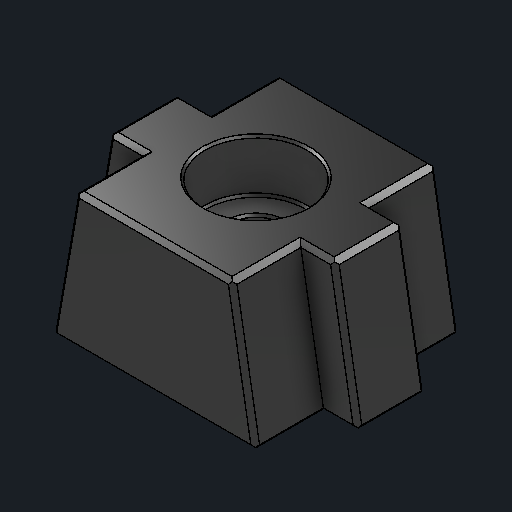
# Autodesk Inventor part: 4 Way Fixture Base
Saved by Autodesk Inventor 2026.2 (Build 302298000, 298)
## iProperties
Created: 2026-05-18
Part Number: 4 Way Fixture Base
Material: ABS Plastic
Document SubType Name: Modeling
Designer: JoshuaEah
Density: 1.06 g/cm^3
Appearance: Glossy - Black
Author: JoshuaEah
Autodesk Inventor part; units mm, degrees
ref_plane "YZ Plane" through (0, 0, 0) normal (1, 0, 0) x (0, 1, 0)
ref_plane "XZ Plane" through (0, 0, 0) normal (0, 1, 0) x (-1, 0, 0)
ref_plane "XY Plane" through (0, 0, 0) normal (0, 0, 1) x (1, 0, 0)
sketch "Sketch4" plane through (0, 0, 0) normal (0, 1, 0) x (-1, 0, 0)
  line L0 (0, 0) -> (-25.4, 0)
  line L1 (-25.4, 0) -> (-25.4, -19.05)
  line L2 (-25.4, -19.05) -> (0, -19.05)
  line L3 (0, -19.05) -> (0, 0)
  line L4 (0, -9.525) -> (-25.4, -9.525) construction
  circle A0 centre (-12.7, -9.525) radius 3.175
  line L5 (-3.175, -19.05) -> (-3.175, 0)
  line L6 (-12.7, -19.05) -> (-12.7, 0) construction
  line L7 (-22.225, -19.05) -> (-22.225, 0)
  line L8 (0, -12.7) -> (-3.175, -12.7)
  line L9 (0, -6.35) -> (-3.175, -6.35)
  line L10 (-25.4, -12.7) -> (-22.225, -12.7)
  line L11 (-25.4, -6.35) -> (-22.225, -6.35)
  point P0 (-25.4, -6.35)
  point P1 (-22.225, -6.35)
  point P2 (-22.225, 0)
  point P3 (-25.4, -12.7)
  point P4 (-22.225, -19.05)
  point P5 (-3.175, -6.35)
  point P6 (0, -6.35)
  dimension "d35" = 25.4
  dimension "d36" = 19.05
  dimension "d37" = 6.35
  dimension "d39" = 3.175
  dimension "d46" = 6.35
  constraints: 24 end point, 8 symmetric about line, 5 midpoint, 4 point on line, 2 horizontal, 2 parallel, 2 perpendicular, 1 centre point, 1 coincident, 1 vertical
  measures "d35" distance of L2.end L1.end
  measures "d36" distance of L1.end L0.end
  measures "d37" diameter of A0
  measures "d39" distance between parallel lines of L3 L5
  measures "d46" diameter of L8 L4
extrude "Extrusion5" add sketch "Sketch4" against normal blind 12.7 contours L3 L9 L5 L0 | L5 L2 L7 L0 | L3 L8 L5 L9 | L7 L11 L1 L0 | L3 L2 L5 L8 | L7 L10 L1 L11 | L7 L2 L1 L10 | A0
extrude "Extrusion6" cut sketch "Sketch4" against normal blind 12.7 contours L3 L9 L5 L0 | L7 L11 L1 L0 | L3 L2 L5 L8 | L7 L2 L1 L10
hole "Hole3" at (12.7, 0, -9.525) direction (0, -1, 0) diameter 5.1054 end through all counterbore diameter 9.525 counterbore depth 4.826 clearance for "Socket Head Cap Screw" size "#10" standard "Ansi Unified Screw Threads"
draft "FaceDraft2" angle 10 pull direction (0, 1, 0) faces at (25.4, -4.2333, -8.4667) (22.225, -4.2333, -16.9333) (22.225, -4.2333, -4.2333) (3.175, -4.2333, -2.1167) (0, -4.2333, -10.5833) (3.175, -4.2333, -14.8167) fixed edges at (25.4, -12.7, -9.525) (22.225, -12.7, -15.875) (22.225, -12.7, -3.175) (3.175, -12.7, -3.175) (3.175, -12.7, -15.875) (0, -12.7, -9.525)
chamfer "Chamfer1" distance 0.4 angle 45 32 edges at (12.7, 0, 0) (2.2394, 0, -9.525) (19.9856, 0, -3.175) (3.8269, 0, -6.35) (5.4144, 0, -3.175) (3.8269, 0, -12.7) (19.9856, 0, -15.875) (5.4144, 0, -15.875) (12.7, 0, -19.05) (21.5731, 0, -12.7) (23.1606, 0, -9.525) (21.5731, 0, -6.35) (3.175, -12.7, -3.175) (1.5875, -12.7, -6.35) (0, -12.7, -9.525) (1.5875, -12.7, -12.7) (3.175, -12.7, -15.875) (12.7, -12.7, -19.05) (22.225, -12.7, -15.875) (23.8125, -12.7, -12.7) (25.4, -12.7, -9.525) (23.8125, -12.7, -6.35) (22.225, -12.7, -3.175) (12.7, -12.7, 0) (1.1197, -6.35, -6.35) (21.1053, -6.35, 0) (4.2947, -6.35, 0) (24.2803, -6.35, -6.35) (24.2803, -6.35, -12.7) (4.2947, -6.35, -19.05) (21.1053, -6.35, -19.05) (1.1197, -6.35, -12.7)
chamfer "Chamfer2" distance 0.2 angle 45 4 edges at (12.7, 0, -14.2875) (12.7, -4.826, -12.0777) (12.7, -4.826, -14.2875) (12.7, -12.7, -12.0777)
body "Solid3"
